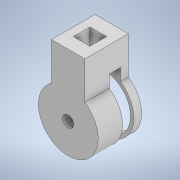
# Autodesk Inventor part: Tilt_Portion
Saved by Autodesk Inventor 2022 (Build 260153000, 153)
## iProperties
Created: 2022-01-01
Part Number: Tilt_Portion
Material: Generic
Document SubType Name: Modeling
Designer: Mlees
Density: 1 g/cm^3
Appearance: Default
Author: Mlees
Autodesk Inventor part; units mm, degrees
ref_plane "YZ Plane" through (0, 0, 0) normal (1, 0, 0) x (0, 1, 0)
ref_plane "XZ Plane" through (0, 0, 0) normal (0, 1, 0) x (-1, 0, 0)
ref_plane "XY Plane" through (0, 0, 0) normal (0, 0, 1) x (1, 0, 0)
sketch "Sketch1" plane through (0, 0, 0) normal (0, 0, 1) x (1, 0, 0)
  circle A0 centre (0, 0) radius 40.5
  arc A1 (-25.4, 37.7504) -> (25.4, 37.7504) centre (0, 0) ccw
  line L0 (-25.4, 37.7504) -> (-25.4, 57.7504)
  line L1 (-25.4, 57.7504) -> (25.4, 57.7504)
  line L2 (25.4, 57.7504) -> (25.4, 37.7504)
  dimension "d1" = 5
  dimension "d9" = 20
  constraints: 6 end point, 2 centre point, 2 perpendicular, 2 point on circle, 1 coincident
  measures "d1" radial gap between concentric circles of A0 A1
  measures "d9" distance of L0.start L0.end
extrude "Extrusion1" add sketch "Sketch1" along normal blind 12
sketch "Sketch2" plane through (-25.4, 57.7504, 0) normal (0, 1, 0) x (1, 0, 0)
  line L0 (0, -12) -> (50.8, -12)
  line L1 (50.8, -12) -> (50.8, 0)
  line L2 (50.8, 0) -> (0, 0)
  line L3 (0, 0) -> (0, -12)
  point P0 (25.4, 0)
  constraints: 8 end point, 2 parallel, 1 horizontal, 1 perpendicular
extrude "Extrusion2" add sketch "Sketch2" along normal blind 12
sketch "Sketch3" plane through (0, 0, 12) normal (0, 0, 1) x (1, 0, 0)
  line L0 (-25.4, 37.7504) -> (-25.4, 69.7504) projected
  line L1 (25.4, 37.7504) -> (25.4, 69.7504) projected
  line L2 (-25.4, 69.7504) -> (25.4, 69.7504)
  line L3 (25.4, 69.7504) -> (25.4, 56.7504)
  line L4 (25.4, 56.7504) -> (-25.4, 56.7504)
  line L5 (-25.4, 56.7504) -> (-25.4, 69.7504)
  point P0 (0, 0)
  dimension "d12" = 13
  constraints: 8 end point, 2 parallel, 1 horizontal, 1 perpendicular, 1 point on line
  measures "d12" distance of L2.end L3.end
extrude "Extrusion3" add sketch "Sketch3" along normal blind 17.2
sketch "Sketch4" plane through (0, 0, 29.2) normal (0, 0, 1) x (1, 0, 0)
  line L0 (25.4, 69.7504) -> (-25.4, 69.7504) projected
  line L1 (-25.4, 69.7504) -> (-25.4, 37.7504)
  circle A0 centre (0, 0) radius 8.5
  arc A1 (-25.4, 37.7504) -> (25.4, 37.7504) centre (0, 0) ccw
  arc A2 (-25.4, 37.7504) -> (25.4, 37.7504) centre (0, 0) ccw projected
  line L2 (25.4, 37.7504) -> (25.4, 69.7504) projected
  line L3 (25.4, 37.7504) -> (25.4, 69.7504)
  line L4 (25.4, 69.7504) -> (-25.4, 69.7504)
  dimension "d15" = 17
  constraints: 6 end point, 2 centre point, 2 coincident, 2 point on circle, 1 collinear, 1 perpendicular
  measures "d15" diameter of A0
extrude "Extrusion4" add sketch "Sketch4" along normal blind 5
sketch "Sketch5" plane through (0, 0, 34.2) normal (0, 0, 1) x (1, 0, 0)
  arc A0 (-25.4, 37.7504) -> (25.4, 37.7504) centre (0, 0) ccw
  circle A1 centre (0, 0) radius 4.5
  line L0 (-25.4, 37.7504) -> (-25.4, 69.7504) projected
  line L1 (-25.4, 37.7504) -> (-25.4, 69.7504)
  line L2 (25.4, 69.7504) -> (-25.4, 69.7504) projected
  line L3 (-25.4, 69.7504) -> (25.4, 69.7504)
  line L4 (25.4, 69.7504) -> (25.4, 37.7504)
  dimension "d18" = 9
  constraints: 6 end point, 2 centre point, 2 coincident, 2 point on circle, 1 collinear, 1 perpendicular, 1 vertical
  measures "d18" diameter of A1
extrude "Extrusion5" add sketch "Sketch5" along normal blind 27
sketch "Sketch6" plane through (0, 0, 61.2) normal (0, 0, 1) x (1, 0, 0)
  line L0 (25.4, 69.7504) -> (-25.4, 69.7504) projected
  line L1 (-25.4, 56.7504) -> (-25.4, 37.7504) projected
  line L2 (-25.4, 69.7504) -> (-25.4, 37.7504)
  line L3 (-25.4, 69.7504) -> (25.4, 69.7504)
  arc A0 (-25.4, 37.7504) -> (25.4, 37.7504) centre (0, 0) ccw projected
  line L4 (25.4, 37.7504) -> (25.4, 69.7504)
  arc A1 (-25.4, 37.7504) -> (25.4, 37.7504) centre (0, 0) ccw
  circle A2 centre (0, 0) radius 8.5
  dimension "d21" = 17
  constraints: 6 end point, 2 centre point, 2 point on circle, 1 coincident, 1 concentric, 1 horizontal, 1 perpendicular, 1 vertical
  measures "d21" diameter of A2
extrude "Extrusion6" add sketch "Sketch6" along normal blind 5
sketch "Sketch7" plane through (-25.4, 69.7504, 0) normal (0, 1, 0) x (1, 0, 0)
  line L0 (50.8, 0) -> (0, 0) projected
  line L1 (0, -29.2) -> (0, -66.2) projected
  line L2 (50.8, 0) -> (0, 0)
  line L3 (0, 0) -> (0, -66.2)
  line L4 (0, -66.2) -> (50.8, -66.2)
  line L5 (50.8, -66.2) -> (50.8, 0)
  point P0 (25.4, 0)
  constraints: 8 end point, 2 parallel, 1 horizontal, 1 perpendicular
extrude "Extrusion7" add sketch "Sketch7" along normal blind 25.4
sketch "Sketch8" plane through (-25.4, 95.1504, 0) normal (0, 1, 0) x (1, 0, 0)
  line L0 (0, -66.2) -> (50.8, -66.2) projected
  line L1 (0, -66.2) -> (50.8, -66.2)
  line L2 (50.8, -66.2) -> (25.4, -66.2)
  line L3 (33.9, -66.2) -> (16.9, -66.2) projected
  line L4 (50.8, -29.2) -> (50.8, -66.2) projected
  line L5 (50.8, 0) -> (50.8, -12) projected
  line L6 (50.8, -66.2) -> (50.8, 0)
  line L7 (50.8, 0) -> (50.8, -33.1)
  line L8 (12.7, -20.4) -> (38.1, -20.4)
  line L9 (38.1, -20.4) -> (38.1, -45.8)
  line L10 (38.1, -45.8) -> (12.7, -45.8)
  line L11 (12.7, -45.8) -> (12.7, -20.4)
  line L12 (43.1, -15.4) -> (7.7, -15.4)
  line L13 (7.7, -15.4) -> (7.7, -50.8)
  line L14 (7.7, -50.8) -> (43.1, -50.8)
  line L15 (43.1, -50.8) -> (43.1, -15.4)
  point P0 (25.4, 0)
  dimension "d30" = 5
  constraints: 24 end point, 4 parallel, 2 horizontal, 2 midpoint, 2 perpendicular, 1 collinear, 3 other
  measures "d30" distance between parallel lines of L8 L12
extrude "Extrusion8" cut sketch "Sketch8" against normal blind 25.4 contours L8 L9 L10 L11
body "Solid1"
